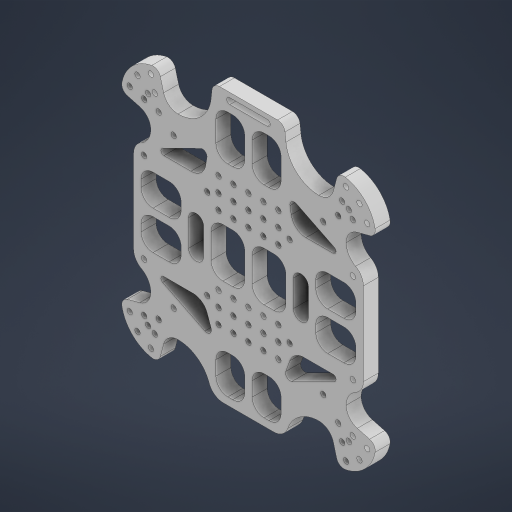
# Autodesk Inventor part: top
Saved by Autodesk Inventor 2023 (Build 270158000, 158)
## iProperties
Created: 2022-06-01
Part Number: top
Material: Generic
Document SubType Name: Modeling
Designer: vibhu
Density: 1 g/cm^3
Appearance: Default
Author: vibhu
Autodesk Inventor part; units mm, degrees
ref_plane "YZ Plane" through (0, 0, 0) normal (1, 0, 0) x (0, 1, 0)
ref_plane "XZ Plane" through (0, 0, 0) normal (0, 1, 0) x (-1, 0, 0)
ref_plane "XY Plane" through (0, 0, 0) normal (0, 0, 1) x (1, 0, 0)
ref_plane "Work Plane1" through (0, 0, 0) normal (0, 0, 1) x (1, 0, 0)
sketch "Sketch1" plane through (0, 0, 0) normal (0, 0, 1) x (1, 0, 0)
  arc A0 (56.7029, -74.1949) -> (47.0436, -66.7831) centre (47.0436, -76.7831) ccw projected
  line L0 (58.9124, -82.4409) -> (56.7029, -74.1949) projected
  arc A1 (58.9124, -82.4409) -> (64.6775, -86.0585) centre (63.742, -81.1468) ccw projected
  arc A2 (64.6775, -86.0585) -> (84.5585, -66.1775) centre (60, -61.5) ccw projected
  arc A3 (84.5585, -66.1775) -> (80.9409, -60.4124) centre (79.6468, -65.242) ccw projected
  line L1 (72.6949, -58.2029) -> (80.9409, -60.4124) projected
  arc A4 (65.2831, -48.5436) -> (72.6949, -58.2029) centre (75.2831, -48.5436) ccw projected
  circle A5 centre (60, -61.5) radius 1.75 projected
  circle A6 centre (67.0711, -68.5711) radius 1.75 projected
  circle A7 centre (62.5882, -71.1593) radius 1.75 projected
  circle A8 centre (69.6593, -64.0882) radius 1.75 projected
  circle A9 centre (79.3185, -66.6764) radius 1.75 projected
  circle A10 centre (74.1421, -75.6421) radius 1.75 projected
  circle A11 centre (65.1764, -80.8185) radius 1.75 projected
  line L2 (-56.7029, -74.1949) -> (-58.9124, -82.4409) projected
  arc A12 (-64.6775, -86.0585) -> (-58.9124, -82.4409) centre (-63.742, -81.1468) ccw projected
  arc A13 (-84.5585, -66.1775) -> (-64.6775, -86.0585) centre (-60, -61.5) ccw projected
  arc A14 (-80.9409, -60.4124) -> (-84.5585, -66.1775) centre (-79.6468, -65.242) ccw projected
  line L3 (-80.9409, -60.4124) -> (-72.6949, -58.2029) projected
  arc A15 (-72.6949, -58.2029) -> (-65.2831, -48.5436) centre (-75.2831, -48.5436) ccw projected
  arc A16 (-47.0436, -66.7831) -> (-56.7029, -74.1949) centre (-47.0436, -76.7831) ccw projected
  circle A17 centre (-62.5882, -71.1593) radius 1.75 projected
  circle A18 centre (-60, -61.5) radius 1.75 projected
  circle A19 centre (-67.0711, -68.5711) radius 1.75 projected
  circle A20 centre (-69.6593, -64.0882) radius 1.75 projected
  circle A21 centre (-79.3185, -66.6764) radius 1.75 projected
  circle A22 centre (-74.1421, -75.6421) radius 1.75 projected
  circle A23 centre (-65.1764, -80.8185) radius 1.75 projected
  arc A24 (-65.2831, 45.5436) -> (-72.6949, 55.2029) centre (-75.2831, 45.5436) ccw projected
  line L4 (-72.6949, 55.2029) -> (-80.9409, 57.4124) projected
  arc A25 (-84.5585, 63.1775) -> (-80.9409, 57.4124) centre (-79.6468, 62.242) ccw projected
  circle A26 centre (-79.3185, 63.6764) radius 1.75 projected
  arc A27 (-64.6775, 83.0585) -> (-84.5585, 63.1775) centre (-60, 58.5) ccw projected
  circle A28 centre (-69.6593, 61.0882) radius 1.75 projected
  circle A29 centre (-60, 58.5) radius 1.75 projected
  circle A30 centre (-67.0711, 65.5711) radius 1.75 projected
  circle A31 centre (-62.5882, 68.1592) radius 1.75 projected
  circle A32 centre (-74.1421, 72.6421) radius 1.75 projected
  circle A33 centre (-65.1764, 77.8185) radius 1.75 projected
  arc A34 (-58.9124, 79.4409) -> (-64.6775, 83.0585) centre (-63.742, 78.1468) ccw projected
  line L5 (-58.9124, 79.4409) -> (-56.7029, 71.1949) projected
  arc A35 (-56.7029, 71.1949) -> (-47.0436, 63.7831) centre (-47.0436, 73.7831) ccw projected
  line L6 (12.5, 86.5) -> (-12.5, 86.5) projected
  arc A36 (12.5, 86.5) -> (12.5, 90.5) centre (12.5, 88.5) ccw projected
  line L7 (-12.5, 90.5) -> (12.5, 90.5) projected
  arc A37 (-12.5, 90.5) -> (-12.5, 86.5) centre (-12.5, 88.5) ccw projected
  line L8 (19.41, 93.5) -> (-19.41, 93.5) projected
  circle A38 centre (-20, 78.5) radius 1.75 construction
  circle A39 centre (-20, 58.5) radius 1.75 construction
  circle A40 centre (20, 58.5) radius 1.75 construction
  circle A41 centre (20, 78.5) radius 1.75 construction
  circle A42 centre (0, 78.5) radius 1.75 construction
  circle A43 centre (0, 58.5) radius 1.75 construction
  arc A44 (47.0436, 63.7831) -> (56.7029, 71.1949) centre (47.0436, 73.7831) ccw projected
  line L9 (56.7029, 71.1949) -> (58.9124, 79.4409) projected
  arc A45 (64.6775, 83.0585) -> (58.9124, 79.4409) centre (63.742, 78.1468) ccw projected
  arc A46 (84.5585, 63.1775) -> (64.6775, 83.0585) centre (60, 58.5) ccw projected
  arc A47 (80.9409, 57.4124) -> (84.5585, 63.1775) centre (79.6468, 62.242) ccw projected
  line L10 (80.9409, 57.4124) -> (72.6949, 55.2029) projected
  arc A48 (72.6949, 55.2029) -> (65.2831, 45.5436) centre (75.2831, 45.5436) ccw projected
  circle A49 centre (60, 58.5) radius 1.75 projected
  circle A50 centre (67.0711, 65.5711) radius 1.75 projected
  circle A51 centre (69.6593, 61.0882) radius 1.75 projected
  circle A52 centre (62.5882, 68.1592) radius 1.75 projected
  circle A53 centre (65.1764, 77.8185) radius 1.75 projected
  circle A54 centre (74.1421, 72.6421) radius 1.75 projected
  circle A55 centre (79.3185, 63.6764) radius 1.75 projected
  circle A56 centre (70, -21.5) radius 1.75 construction
  circle A57 centre (50, -21.5) radius 1.75 construction
  circle A58 centre (50, 18.5) radius 1.75 construction
  circle A59 centre (60, 18.5) radius 1.75 construction
  circle A60 centre (-50, 18.5) radius 1.75 construction
  circle A61 centre (-70, 18.5) radius 1.75 construction
  circle A62 centre (-70, -21.5) radius 1.75 construction
  circle A63 centre (-50, -21.5) radius 1.75 construction
  circle A64 centre (-70, -1.5) radius 1.75 construction
  circle A65 centre (-50, -1.5) radius 1.75 construction
  circle A66 centre (-20, -11.5) radius 1.75 construction
  circle A67 centre (-20, 8.5) radius 1.75 construction
  circle A68 centre (20, 8.5) radius 1.75 construction
  circle A69 centre (20, -11.5) radius 1.75 construction
  circle A70 centre (0, -11.5) radius 1.75 construction
  circle A71 centre (0, 8.5) radius 1.75 construction
  circle A72 centre (-27.5, -31.5) radius 1.75 projected
  circle A73 centre (-27.5, 28.5) radius 1.75 projected
  circle A74 centre (27.5, -31.5) radius 1.75 projected
  circle A75 centre (27.5, 28.5) radius 1.75 projected
  circle A76 centre (-20, -61.5) radius 1.75 construction
  circle A77 centre (20, -61.5) radius 1.75 construction
  circle A78 centre (0, -61.5) radius 1.75 construction
  circle A79 centre (0, -81.5) radius 1.75 construction
  circle A80 centre (20, -81.5) radius 1.75 construction
  circle A81 centre (-20, -81.5) radius 1.75 construction
  arc A82 (-71.5515, 34.9664) -> (-65.2831, 45.5436) centre (-77.3412, 45.5436) ccw projected
  arc A83 (-71.5515, 34.9664) -> (-76.75, 26.1945) centre (-66.75, 26.1945) ccw projected
  line L11 (-76.75, 26.1945) -> (-76.75, -29.1946) projected
  arc A84 (-76.75, -29.1946) -> (-71.5515, -37.9664) centre (-66.75, -29.1946) ccw projected
  arc A85 (-65.2831, -48.5436) -> (-71.5515, -37.9664) centre (-77.3412, -48.5436) ccw projected
  arc A86 (-26.2294, -81.5524) -> (-47.0436, -66.7831) centre (-47.0436, -88.8345) ccw projected
  arc A87 (-26.2294, -81.5524) -> (-16.7904, -88.25) centre (-16.7904, -78.25) ccw projected
  line L12 (-16.7904, -88.25) -> (16.7904, -88.25) projected
  arc A88 (16.7904, -88.25) -> (26.2294, -81.5524) centre (16.7904, -78.25) ccw projected
  arc A89 (47.0436, -66.7831) -> (26.2294, -81.5524) centre (47.0436, -88.8345) ccw projected
  arc A90 (71.5515, -37.9664) -> (65.2831, -48.5436) centre (77.3412, -48.5436) ccw projected
  arc A91 (71.5515, -37.9664) -> (76.75, -29.1946) centre (66.75, -29.1946) ccw projected
  line L13 (76.75, -29.1946) -> (76.75, 26.1945) projected
  arc A92 (76.75, 26.1945) -> (71.5515, 34.9664) centre (66.75, 26.1945) ccw projected
  arc A93 (65.2831, 45.5436) -> (71.5515, 34.9664) centre (77.3412, 45.5436) ccw projected
  arc A94 (25, 83.5) -> (47.0436, 63.7831) centre (47.0436, 85.964) ccw projected
  line L14 (25, 83.5) -> (24.379, 89.0554) projected
  arc A95 (24.379, 89.0554) -> (19.41, 93.5) centre (19.41, 88.5) ccw projected
  arc A96 (-19.41, 93.5) -> (-24.379, 89.0554) centre (-19.41, 88.5) ccw projected
  line L15 (-24.379, 89.0554) -> (-25, 83.5) projected
  arc A97 (-47.0436, 63.7831) -> (-25, 83.5) centre (-47.0436, 85.964) ccw projected
  circle A98 centre (-69.75, 28.5) radius 1.75 projected
  circle A99 centre (-69.75, -31.5) radius 1.75 projected
  circle A100 centre (69.75, -31.5) radius 1.75 projected
  circle A101 centre (69.75, 28.5) radius 1.75 projected
  arc A102 (-30, 7.3197) -> (-40, 7.3197) centre (-35, 7.3197) ccw projected
  line L16 (-40, -10.3197) -> (-40, 7.3197) projected
  arc A103 (-40, -10.3197) -> (-30, -10.3197) centre (-35, -10.3197) ccw projected
  line L17 (-30, 7.3197) -> (-30, -10.3197) projected
  line L18 (30, -10.3197) -> (30, 7.3197) projected
  arc A104 (40, 7.3197) -> (30, 7.3197) centre (35, 7.3197) ccw projected
  line L19 (40, 7.3197) -> (40, -10.3197) projected
  arc A105 (30, -10.3197) -> (40, -10.3197) centre (35, -10.3197) ccw projected
  line L20 (0, 103.8322) -> (0, -136.6976) construction
  circle A106 centre (-20, 21.5902) radius 1.75
  line L21 (0, -95.4139) -> (24.379, -95.4139) construction
  circle A107 centre (-20, 31.5902) radius 1.75
  circle A108 centre (-20, 41.5902) radius 1.75
  circle A109 centre (-10, 21.5902) radius 1.75
  circle A110 centre (-10, 31.5902) radius 1.75
  circle A111 centre (-10, 41.5902) radius 1.75
  circle A112 centre (0, 21.5902) radius 1.75
  circle A113 centre (0, 31.5902) radius 1.75
  circle A114 centre (0, 41.5902) radius 1.75
  circle A115 centre (10, 21.5902) radius 1.75
  circle A116 centre (10, 31.5902) radius 1.75
  circle A117 centre (10, 41.5902) radius 1.75
  circle A118 centre (20, 21.5902) radius 1.75
  circle A119 centre (20, 31.5902) radius 1.75
  circle A120 centre (20, 41.5902) radius 1.75
  line L22 (-5, 34.0902) -> (-35.7042, 34.0902) construction
  line L23 (-36.5279, 29.0902) -> (-8, 29.0902) construction
  line L24 (-15.4957, 34.0902) -> (-15.4957, 29.0902) construction
  circle A121 centre (-20, -24.5902) radius 1.75
  circle A122 centre (-20, -34.5902) radius 1.75
  circle A123 centre (-20, -44.5902) radius 1.75
  circle A124 centre (-10, -24.5902) radius 1.75
  circle A125 centre (-10, -34.5902) radius 1.75
  circle A126 centre (-10, -44.5902) radius 1.75
  circle A127 centre (0, -24.5902) radius 1.75
  circle A128 centre (0, -34.5902) radius 1.75
  circle A129 centre (0, -44.5902) radius 1.75
  circle A130 centre (10, -24.5902) radius 1.75
  circle A131 centre (10, -34.5902) radius 1.75
  circle A132 centre (10, -44.5902) radius 1.75
  circle A133 centre (20, -24.5902) radius 1.75
  circle A134 centre (20, -34.5902) radius 1.75
  circle A135 centre (20, -44.5902) radius 1.75
  line L25 (-8, -32.0902) -> (-36.5279, -32.0902) construction
  line L26 (-35.7042, -37.0902) -> (-5, -37.0902) construction
  line L27 (-15.1289, -32.0902) -> (-15.1289, -37.0902) construction
  point P0 (0, 0)
  point P1 (-76.75, -1.5)
  point P2 (-15.4957, 31.5902)
  point P3 (-15.1289, -34.5902)
  dimension "d6" = 3.5
  dimension "d9" = 10
  dimension "d12" = 10
  dimension "d17" = 10
  dimension "d20" = 10
  constraints: 30 centre point, 12 end point, 6 point on line, 5 horizontal, 3 midpoint, 3 vertical, 2 horizontal alignment, 2 perpendicular, 2 vertical alignment, 1 equal radius, 60 other
  measures "d6" diameter of A106
  measures "d9" distance of A106.centre A107.centre
  measures "d12" distance of A106.centre A109.centre
  measures "d17" distance of A121.centre A122.centre
  measures "d20" distance of A121.centre A124.centre
extrude "Extrusion1" add sketch "Sketch1" along normal blind 10
sketch "Sketch2" plane through (0, 0, 10) normal (0, 0, 1) x (1, 0, 0)
  circle A0 centre (-20, -61.5) radius 1.75 construction
  circle A1 centre (-20, -81.5) radius 1.75 construction
  circle A2 centre (20, -81.5) radius 1.75 construction
  circle A3 centre (20, -61.5) radius 1.75 construction
  circle A4 centre (50, -21.5) radius 1.75 construction
  circle A5 centre (70, -21.5) radius 1.75 construction
  circle A6 centre (50, 18.5) radius 1.75 construction
  circle A7 centre (-70, 18.5) radius 1.75 construction
  circle A8 centre (-50, 18.5) radius 1.75 construction
  circle A9 centre (-70, -21.5) radius 1.75 construction
  circle A10 centre (-50, -21.5) radius 1.75 construction
  circle A11 centre (-20, 58.5) radius 1.75 construction
  circle A12 centre (20, 58.5) radius 1.75 construction
  circle A13 centre (20, 78.5) radius 1.75 construction
  circle A14 centre (-20, 78.5) radius 1.75 construction
  circle A15 centre (-20, -11.5) radius 1.75 construction
  circle A16 centre (20, -11.5) radius 1.75 construction
  circle A17 centre (20, 8.5) radius 1.75 construction
  circle A18 centre (-20, 8.5) radius 1.75 construction
  line L0 (-71.75, 21.75) -> (-45, 21.75)
  line L1 (-45, 21.75) -> (-45, -24.75)
  line L2 (-45, -24.75) -> (-71.75, -24.75)
  line L3 (-71.75, -24.75) -> (-71.75, 21.75)
  line L4 (-76.75, 26.1945) -> (-76.75, -29.1946) projected
  circle A19 centre (-69.75, 28.5) radius 1.75 projected
  line L5 (-40, -10.3197) -> (-40, 7.3197) projected
  line L6 (-71.75, 1) -> (-45, 1)
  line L7 (-45, 1) -> (-45, -4)
  line L8 (-45, -4) -> (-71.75, -4)
  line L9 (-71.75, -4) -> (-71.75, 1)
  line L10 (-25, 14.8402) -> (25, 14.8402)
  line L11 (25, 14.8402) -> (25, -17.8402)
  line L12 (25, -17.8402) -> (-25, -17.8402)
  line L13 (-25, -17.8402) -> (-25, 14.8402)
  line L14 (-30, 7.3197) -> (-30, -10.3197) projected
  line L15 (30, -10.3197) -> (30, 7.3197) projected
  circle A20 centre (-20, 21.5902) radius 1.75 construction
  circle A21 centre (-20, -24.5902) radius 1.75 construction
  line L16 (-2.5, 14.8402) -> (2.5, 14.8402)
  line L17 (2.5, 14.8402) -> (2.5, -17.8402)
  line L18 (2.5, -17.8402) -> (-2.5, -17.8402)
  line L19 (-2.5, -17.8402) -> (-2.5, 14.8402)
  line L20 (0, 120.2032) -> (0, -113.5378) construction
  line L21 (-21.75, 81.5) -> (21.75, 81.5)
  line L22 (21.75, 81.5) -> (21.75, 51.5902)
  line L23 (21.75, 51.5902) -> (-21.75, 51.5902)
  line L24 (-21.75, 51.5902) -> (-21.75, 81.5)
  line L25 (-2.5, 81.5) -> (2.5, 81.5)
  line L26 (2.5, 81.5) -> (2.5, 51.5902)
  line L27 (2.5, 51.5902) -> (-2.5, 51.5902)
  line L28 (-2.5, 51.5902) -> (-2.5, 81.5)
  line L29 (12.5, 86.5) -> (-12.5, 86.5) projected
  circle A22 centre (-20, 41.5902) radius 1.75 projected
  line L30 (0, 0) -> (110.9609, 0) construction
  circle A23 centre (70, 18.5) radius 1.75 construction
  circle A24 centre (50, 18.5) radius 1.75 construction
  circle A25 centre (70, -21.5) radius 1.75 construction
  circle A26 centre (50, -21.5) radius 1.75 construction
  line L31 (71.75, 21.75) -> (45, 21.75)
  line L32 (45, 21.75) -> (45, -24.75)
  line L33 (45, -24.75) -> (71.75, -24.75)
  line L34 (71.75, -24.75) -> (71.75, 21.75)
  line L35 (71.75, 1) -> (45, 1)
  line L36 (45, 1) -> (45, -4)
  line L37 (45, -4) -> (71.75, -4)
  line L38 (71.75, -4) -> (71.75, 1)
  line L39 (-21.75, -57.75) -> (21.75, -57.75)
  line L40 (21.75, -57.75) -> (21.75, -83.25)
  line L41 (21.75, -83.25) -> (-21.75, -83.25)
  line L42 (-21.75, -83.25) -> (-21.75, -57.75)
  line L43 (-2.5, -57.75) -> (2.5, -57.75)
  line L44 (2.5, -57.75) -> (2.5, -83.25)
  line L45 (2.5, -83.25) -> (-2.5, -83.25)
  line L46 (-2.5, -83.25) -> (-2.5, -57.75)
  line L47 (-16.7904, -88.25) -> (16.7904, -88.25) projected
  point P0 (-40, -1.5)
  point P1 (-45, -1.5)
  point P2 (-45, -1.5)
  point P3 (0, 14.8402)
  point P4 (0, 14.8402)
  point P5 (0, 81.5)
  point P6 (0, 81.5)
  point P7 (45, -1.5)
  point P8 (45, -1.5)
  point P9 (0, -57.75)
  point P10 (0, -57.75)
  point P11 (2.5, 81.5)
  point P12 (2.5, 51.5902)
  point P13 (-2.5, 81.5)
  point P14 (-2.5, -83.25)
  point P15 (2.5, -17.8402)
  dimension "d25" = 5
  dimension "d27" = 5
  dimension "d28" = 5
  dimension "d29" = 5
  dimension "d30" = 5
  dimension "d31" = 5
  dimension "d33" = 5
  dimension "d34" = 5
  dimension "d35" = 5
  dimension "d36" = 5
  dimension "d37" = 10
  dimension "d38" = 5
  dimension "d40" = 5
  dimension "d41" = 5
  dimension "d42" = 2
  constraints: 84 end point, 16 parallel, 14 symmetric about line, 9 horizontal, 9 midpoint, 8 collinear, 8 perpendicular, 4 centre point, 4 coincident, 3 point on line, 2 tangent, 1 horizontal alignment, 1 vertical, 4 other
  measures "d25" distance between parallel lines of L4 L3
  measures "d27" distance edge to line of A19 L0
  measures "d28" distance between parallel lines of L5 L1
  measures "d29" distance between parallel lines of L8 L6
  measures "d30" distance between parallel lines of L13 L14
  measures "d31" distance between parallel lines of L15 L11
  measures "d33" distance edge to line of A20 L10
  measures "d34" distance edge to line of A21 L12
  measures "d35" distance between parallel lines of L17 L19
  measures "d36" distance between parallel lines of L21 L29
  measures "d37" distance from line of A22.centre L23
  measures "d38" distance between parallel lines of L26 L28
  measures "d40" distance between parallel lines of L44 L46
  measures "d41" distance between parallel lines of L41 L47
  measures "d42" distance edge to line of A0 L39
extrude "Extrusion2" cut sketch "Sketch2" against normal up to surface (10 mm away) contours L0 L1 L6 L3 | L8 L1 L2 L3 | L10 L19 L12 L13 | L10 L11 L12 L17 | L21 L28 L23 L24 | L21 L22 L23 L26 | L34 L35 L32 L31 | L34 L33 L32 L37 | L39 L46 L41 L42 | L39 L40 L41 L44
fillet "Fillet1" radius 8 40 edges at (-45, -24.75, 5) (-45, -4, 5) (-45, 21.75, 5) (-45, 1, 5) (-71.75, 21.75, 5) (-71.75, 1, 5) (-71.75, -4, 5) (-71.75, -24.75, 5) (-21.75, -57.75, 5) (-2.5, -57.75, 5) (2.5, -57.75, 5) (21.75, -57.75, 5) (21.75, -83.25, 5) (2.5, -83.25, 5) (-2.5, -83.25, 5) (-21.75, -83.25, 5) (-2.5, 14.8402, 5) (-25, 14.8402, 5) (-25, -17.8402, 5) (-2.5, -17.8402, 5) (2.5, -17.8402, 5) (2.5, 14.8402, 5) (25, 14.8402, 5) (25, -17.8402, 5) (71.75, 21.75, 5) (71.75, 1, 5) (71.75, -4, 5) (71.75, -24.75, 5) (45, -24.75, 5) (45, -4, 5) (45, 1, 5) (45, 21.75, 5) (-2.5, 51.5902, 5) (2.5, 51.5902, 5) (2.5, 81.5, 5) (-2.5, 81.5, 5) (-21.75, 81.5, 5) (-21.75, 51.5902, 5) (21.75, 81.5, 5) (21.75, 51.5902, 5)
sketch "Sketch3" plane through (0, 0, 10) normal (0, 0, 1) x (1, 0, 0)
  line L0 (-50, 50) -> (50, 50) construction
  line L1 (50, 50) -> (50, -50) construction
  line L2 (50, -50) -> (-50, -50) construction
  line L3 (-50, -50) -> (-50, 50) construction
  line L4 (-50, 50) -> (50, -50) construction
  line L5 (50, 50) -> (-50, -50) construction
  circle A0 centre (-50, 50) radius 1.75
  circle A1 centre (50, 50) radius 1.75
  circle A2 centre (50, -50) radius 1.75
  circle A3 centre (-50, -50) radius 1.75
  point P0 (0, 0)
  dimension "d46" = 100
  dimension "d47" = 100
  dimension "d48" = 3.5
  constraints: 12 end point, 4 centre point, 4 coincident, 3 equal radius, 2 midpoint, 2 parallel, 1 horizontal, 1 perpendicular
  measures "d46" distance of L1.end L2.end
  measures "d47" distance of L0.end L1.end
  measures "d48" diameter of A0
extrude "Extrusion3" cut sketch "Sketch3" against normal up to surface (10 mm away)
sketch "Sketch4" plane through (0, 0, 0) normal (0, 0, -1) x (-1, 0, 0)
  circle A0 centre (-20, 41.5902) radius 1.75 construction
  circle A1 centre (-20, 41.5902) radius 3.25
  circle A2 centre (-20, -24.5902) radius 1.75 construction
  circle A3 centre (-20, -24.5902) radius 3.25
  line L0 (0, 0) -> (22.8644, 0) construction
  line L1 (22.8644, 0) -> (0, 0)
  line L2 (0, 16.9905) -> (0, 0) construction
  circle A4 centre (-10, -24.5902) radius 3.25
  circle A5 centre (0, -24.5902) radius 3.25
  circle A6 centre (10, -24.5902) radius 3.25
  circle A7 centre (20, -24.5902) radius 3.25
  circle A8 centre (-20, -34.5902) radius 3.25
  circle A9 centre (-10, -34.5902) radius 3.25
  circle A10 centre (0, -34.5902) radius 3.25
  circle A11 centre (10, -34.5902) radius 3.25
  circle A12 centre (20, -34.5902) radius 3.25
  circle A13 centre (-20, -44.5902) radius 3.25
  circle A14 centre (-10, -44.5902) radius 3.25
  circle A15 centre (0, -44.5902) radius 3.25
  circle A16 centre (10, -44.5902) radius 3.25
  circle A17 centre (20, -44.5902) radius 3.25
  circle A18 centre (-10, 41.5902) radius 3.25
  circle A19 centre (0, 41.5902) radius 3.25
  circle A20 centre (10, 41.5902) radius 3.25
  circle A21 centre (20, 41.5902) radius 3.25
  circle A22 centre (-20, 31.5902) radius 3.25
  circle A23 centre (-10, 31.5902) radius 3.25
  circle A24 centre (0, 31.5902) radius 3.25
  circle A25 centre (10, 31.5902) radius 3.25
  circle A26 centre (20, 31.5902) radius 3.25
  circle A27 centre (-20, 21.5902) radius 3.25
  circle A28 centre (-10, 21.5902) radius 3.25
  circle A29 centre (0, 21.5902) radius 3.25
  circle A30 centre (10, 21.5902) radius 3.25
  circle A31 centre (20, 21.5902) radius 3.25
  dimension "d51" = 6.5
  dimension "d52" = 6.5
  dimension "d60" = 10
  dimension "d63" = 10
  dimension "d68" = 10
  dimension "d71" = 10
  constraints: 30 centre point, 6 end point, 3 horizontal, 2 coincident, 2 vertical, 1 collinear, 1 perpendicular, 56 other
  measures "d51" diameter of A1
  measures "d52" diameter of A3
  measures "d60" distance of A3.centre A4.centre
  measures "d63" distance of A3.centre A8.centre
  measures "d68" distance of A1.centre A18.centre
  measures "d71" distance of A1.centre A22.centre
extrude "Extrusion4" cut sketch "Sketch4" against normal blind 3
sketch "Sketch5" plane through (0, 0, 10) normal (0, 0, 1) x (1, 0, 0)
  line L0 (-65, 35) -> (-30, 35)
  line L1 (-30, 35) -> (-26.75, 54.0258)
  line L2 (-26.75, 54.0258) -> (-65, 35)
  line L3 (26.75, 54.0258) -> (30, 35)
  line L4 (30, 35) -> (65, 35)
  line L5 (65, 35) -> (26.75, 54.0258)
  line L6 (30, -35) -> (65, -35)
  line L7 (65, -35) -> (22.4805, -56.1495)
  line L8 (22.4805, -56.1495) -> (30, -35)
  line L9 (-65, -35) -> (-30, -35)
  line L10 (-30, -35) -> (-22.4805, -56.1495)
  line L11 (-22.4805, -56.1495) -> (-65, -35)
  line L12 (-30, -35) -> (30, -35) construction
  line L13 (30, -35) -> (30, 35) construction
  line L14 (30, 35) -> (-30, 35) construction
  line L15 (-30, 35) -> (-30, -35) construction
  line L16 (-30, -35) -> (30, 35) construction
  line L17 (30, -35) -> (-30, 35) construction
  line L18 (-22.4805, -56.1495) -> (22.4805, -56.1495) construction
  line L19 (-26.75, 54.0258) -> (26.75, 54.0258) construction
  line L20 (-21.75, 59.5902) -> (-21.75, 73.5) projected
  circle A0 centre (-50, 50) radius 1.75 projected
  circle A1 centre (-50, -50) radius 1.75 projected
  arc A2 (-13.75, -57.75) -> (-21.75, -65.75) centre (-13.75, -65.75) ccw projected
  point P0 (0, 0)
  point P1 (0, -35)
  point P2 (0, -56.1495)
  point P3 (0, 54.0258)
  point P4 (0, 35)
  point P5 (-19.4069, -60.0932)
  dimension "d76" = 70
  dimension "d77" = 5
  dimension "d78" = 5
  dimension "d79" = 5
  dimension "d80" = 35
  dimension "d81" = 60
  dimension "d82" = 5
  constraints: 41 end point, 6 midpoint, 5 vertical alignment, 4 horizontal, 3 equal length, 2 collinear, 2 horizontal alignment, 2 point on line, 1 perpendicular, 1 point on circle
  measures "d76" distance of L0.end L12.start
  measures "d77" distance from line of L20 L1.end
  measures "d78" distance edge to line of A0 L2
  measures "d79" distance edge to line of A1 L11
  measures "d80" distance of L0.start L0.end
  measures "d81" distance of L3.end L0.end
  measures "d82" distance of point (-19.407, -60.093) L10.end
extrude "Extrusion5" cut sketch "Sketch5" against normal up to surface (10 mm away) contours L2 L1 L0 | L5 L4 L3 | L6 L7 L8 | L9 L10 L11
fillet "Fillet2" radius 3 4 edges at (26.75, 54.0258, 5) (-26.75, 54.0258, 5) (-22.4805, -56.1495, 5) (22.4805, -56.1495, 5)
fillet "Fillet3" radius 10 4 edges at (30, -35, 5) (30, 35, 5) (-30, 35, 5) (-30, -35, 5)
fillet "Fillet4" radius 2 4 edges at (65, 35, 5) (65, -35, 5) (-65, -35, 5) (-65, 35, 5)
body "Solid1"
